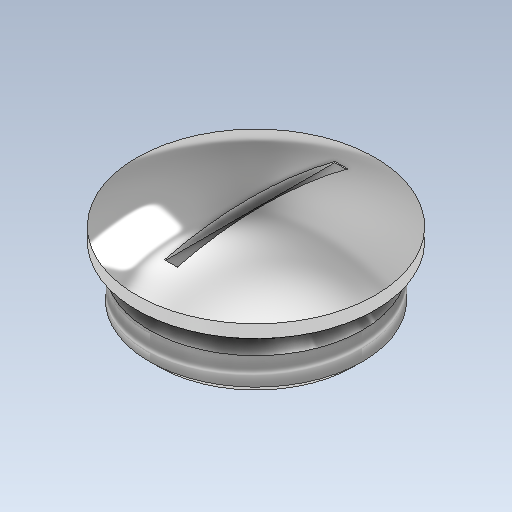
# Autodesk Inventor part: Cartridge Glans Cover RS 406-9413 LAPP
Saved by Autodesk Inventor 2021 (Build 250183000, 183)
## iProperties
Created: 2020-05-01
Part Number: Cartridge Glans Cover RS 406-9413 LAPP
Material: Generic
Document SubType Name: Modeling
Designer: jgray
Density: 1 g/cm^3
Appearance: Chrome - Polished
Author: jgray
Autodesk Inventor part; units mm, degrees
ref_plane "YZ Plane" through (0, 0, 0) normal (1, 0, 0) x (0, 1, 0)
ref_plane "XZ Plane" through (0, 0, 0) normal (0, 1, 0) x (-1, 0, 0)
ref_plane "XY Plane" through (0, 0, 0) normal (0, 0, 1) x (1, 0, 0)
sketch "Sketch1" plane through (0, 0, 0) normal (0, 1, 0) x (-1, 0, 0)
  circle A0 centre (0, 0) radius 14
  dimension "d0" = 28
  constraints: 1 centre point, 1 coincident
  measures "d0" diameter of A0
extrude "Extrusion1" add sketch "Sketch1" along normal blind 1.5
sketch "Sketch2" plane through (0, 0, 0) normal (0, -1, 0) x (1, 0, 0)
  circle A0 centre (0, 0) radius 11
  dimension "d3" = 22
  constraints: 1 centre point, 1 coincident
  measures "d3" diameter of A0
extrude "Extrusion2" add sketch "Sketch2" along normal blind 1.8
sketch "Sketch3" plane through (0, -1.8, 0) normal (0, -1, 0) x (1, 0, 0)
  circle A0 centre (0, 0) radius 12.5
  dimension "d6" = 25
  constraints: 1 centre point, 1 coincident
  measures "d6" diameter of A0
extrude "Extrusion3" add sketch "Sketch3" along normal blind 5.2
chamfer "Chamfer1" distance 1 angle 45 2 edges at (-12.5, -1.8, 0) (-12.5, -7, 0)
thread "Thread1" size "M25x2" class "6g" standard "ANSI Metric M Profile" full length
sketch "Sketch4" plane through (0, 0, 0) normal (0, 0, 1) x (1, 0, 0)
  line L0 (0, 11.1309) -> (0, -17.3821)
  line L1 (14, 1.5) -> (-14, 1.5) projected
  circle A0 centre (0, -36.45) radius 40.45
  line L2 (11.5, -7) -> (-11.5, -7) projected
  point P0 (0, 0)
  point P1 (0, 4)
  point P2 (0, 1.5)
  dimension "d15" = 11
  constraints: 2 end point, 2 point on line, 1 vertical, 3 other
revolve "Revolution1" add sketch "Sketch4" angle 360 about axis through (0, 11.1309, 0) along (0, -1, 0) picked at (7.8142, 1.9608) contours A0 L1 L0
sketch "Sketch5" plane through (0, 0, 0) normal (0, 0, 1) x (1, 0, 0)
  line L0 (-0.75, 5.2944) -> (-0.75, 2.6153)
  line L1 (-0.75, 2.6153) -> (0.75, 2.6153)
  line L2 (0.75, 2.6153) -> (0.75, 5.2944)
  line L3 (0.75, 5.2944) -> (-0.75, 5.2944)
  line L4 (-0.75, 5.2944) -> (0.75, 2.6153) construction
  line L5 (-0.75, 2.6153) -> (0.75, 5.2944) construction
  point P0 (0, 0)
  point P1 (0, 3.9548)
  dimension "d17" = 1.5
  constraints: 12 end point, 2 midpoint, 2 parallel, 1 perpendicular, 1 vertical
  measures "d17" distance of L1.end L0.end
extrude "Extrusion4" cut sketch "Sketch5" against normal mid plane 20
sketch "Sketch6" plane through (0, -7, 0) normal (0, -1, 0) x (1, 0, 0)
  circle A0 centre (0, 0) radius 10
  dimension "d20" = 20
  constraints: 1 centre point, 1 coincident
  measures "d20" diameter of A0
extrude "Extrusion5" cut sketch "Sketch6" against normal blind 7.5
chamfer "Chamfer2" distance 0.5 angle 45 2 edges at (-10, 0.5, 0) (-10, -7, 0)
body "Solid1"
